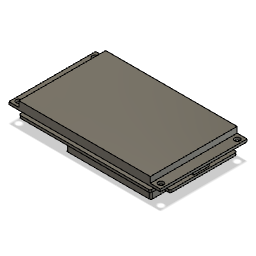
FreeTouchDeck Case V1 (Autodesk Fusion 360 archive; units mm, degrees)
design "ILI9488 TFT"
Autodesk Fusion 360 part; units mm, degrees
sketch "TFT_PCB" plane through (0, 0, 0) normal (0, 1, 0) x (1, 0, 0)
  line L0 (49.15, -28.17) -> (-49.15, -28.17)
  line L1 (-49.15, -28.17) -> (-49.15, 28.17)
  line L2 (-49.15, 28.17) -> (49.15, 28.17)
  line L3 (49.15, 28.17) -> (49.15, -28.17)
  line L4 (49.15, -28.17) -> (-49.15, 28.17) construction
  line L5 (-49.15, -28.17) -> (49.15, 28.17) construction
  line L6 (-42.65, 28.17) -> (-42.65, -28.17)
  line L7 (42.65, 28.17) -> (42.65, -28.17)
  circle A0 centre (-46.15, 24.75) radius 1.75
  line L8 (0, 28.17) -> (0, -28.17) construction
  line L9 (-49.15, 0) -> (49.15, 0) construction
  circle A1 centre (46.15, 24.75) radius 1.75
  circle A2 centre (-46.15, -24.75) radius 1.75
  circle A3 centre (46.15, -24.75) radius 1.75
  dimension "d4" = 98.3
  dimension "d5" = 56.34
  dimension "d6" = 6.5
  dimension "d7" = 6.5
  dimension "d8" = 3.5
  dimension "d9" = 3.42
  dimension "d10" = 3
  constraint horizontal L0
  constraint perpendicular L0 L1
  constraint parallel L0 L2
  constraint parallel L1 L3
  constraint coincident L4 origin
  constraint coincident L5 origin
  constraint coincident L2 L6.start
  constraint coincident L0 L6.end
  constraint perpendicular L0 L6
  constraint coincident L2 L7.start
  constraint coincident L0 L7.end
  constraint perpendicular L0 L7
  constraint midpoint L2 L8.start
  constraint midpoint L0 L8.end
  constraint midpoint L1 L9.start
  constraint midpoint L3 L9.end
  constraint symmetric A0 L8 A1
  constraint symmetric A0 L9 A2
  constraint symmetric L9 A1 A3
  measures "d4" distance of L1.end L2.end
  measures "d5" distance of L0.end L1.end
  measures "d6" distance of L1 L6
  measures "d7" distance of L3 L7
  measures "d8" diameter of A0
  measures "d9" distance of L2 A0.centre
  measures "d10" distance of L1 A0.centre
extrude "Extrude1" add sketch "TFT_PCB" against normal blind 1.6 makes body 1
extrude "Extrude2" add sketch "TFT_PCB" along normal blind 3.79 contours L0 L2 L6 L7 bodies 1
sketch "Sketch2" plane through (0, -1.6, 0) normal (0, -1, 0) x (1, 0, 0)
  circle A0 centre (-46.15, 24.75) radius 1.75
  circle A1 centre (46.15, -24.75) radius 1.75
  circle A2 centre (46.15, 24.75) radius 1.75
  circle A3 centre (-46.15, -24.75) radius 1.75
  line L0 (-49.15, -28.17) -> (49.15, -28.17)
  line L1 (49.15, -28.17) -> (49.15, 28.17)
  line L2 (49.15, 28.17) -> (-49.15, 28.17)
  line L3 (-49.15, 28.17) -> (-49.15, -28.17)
  line L4 (-48.13, 17.69) -> (-45.98, 17.69)
  line L5 (-45.98, 17.69) -> (-45.98, -17.97)
  line L6 (-45.98, -17.97) -> (-48.13, -17.97)
  line L7 (-48.13, -17.97) -> (-48.13, 17.69)
  line L8 (45.98, 5.73) -> (48.13, 5.73)
  line L9 (48.13, 5.73) -> (48.13, -4.67)
  line L10 (48.13, -4.67) -> (45.98, -4.67)
  line L11 (45.98, -4.67) -> (45.98, 5.73)
  dimension "d15" = 2.15
  dimension "d16" = 35.66
  dimension "d17" = 10.2
  dimension "d18" = 1.02
  dimension "d19" = 2.15
  dimension "d20" = 10.4
  dimension "d21" = 1.02
  dimension "d22" = 23.5
  constraint horizontal L4
  constraint vertical L5
  constraint horizontal L6
  constraint vertical L7
  constraint horizontal L8
  constraint vertical L9
  constraint horizontal L10
  constraint vertical L11
  measures "d15" distance of L4.start L4.end
  measures "d16" distance of L4.start L6.end
  measures "d17" distance of L0 L6
  measures "d18" distance of L3 L7
  measures "d19" distance of L8.start L8.end
  measures "d20" distance of L8.start L10.end
  measures "d21" distance of L1 L9
  measures "d22" distance of L0 L10
extrude "Extrude3" add sketch "Sketch2" along normal blind 2.4 contours L4 L5 L6 L7 | L8 L9 L10 L11 bodies 1
sketch "Sketch3" plane through (0, -4, 0) normal (0, -1, 0) x (1, 0, 0)
  line L0 (-48.13, -17.97) -> (-45.98, -17.97)
  line L1 (-45.98, -17.97) -> (-45.98, 17.69)
  line L2 (-45.98, 17.69) -> (-48.13, 17.69)
  line L3 (-48.13, 17.69) -> (-48.13, -17.97)
  line L4 (45.98, -4.67) -> (45.98, 5.73)
  line L5 (45.98, 5.73) -> (48.13, 5.73)
  line L6 (48.13, 5.73) -> (48.13, -4.67)
  line L7 (48.13, -4.67) -> (45.98, -4.67)
  line L8 (-48.13, -17.97) -> (-48.13, 17.69)
  line L9 (-48.13, 17.69) -> (-45.98, 17.69)
  line L10 (-45.98, 17.69) -> (-45.98, -17.97)
  line L11 (-45.98, -17.97) -> (-48.13, -17.97)
  circle A0 centre (-46.15, 24.75) radius 1.75
  circle A1 centre (46.15, -24.75) radius 1.75
  circle A2 centre (46.15, 24.75) radius 1.75
  circle A3 centre (-46.15, -24.75) radius 1.75
  line L12 (-49.15, -28.17) -> (49.15, -28.17)
  line L13 (49.15, -28.17) -> (49.15, 28.17)
  line L14 (49.15, 28.17) -> (-49.15, 28.17)
  line L15 (-49.15, 28.17) -> (-49.15, -28.17)
  line L16 (-49.15, 28.17) -> (-42.65, 28.17)
  line L17 (-42.65, 28.17) -> (-42.65, 21.67)
  line L18 (-42.65, 21.67) -> (-49.15, 21.67)
  line L19 (-49.15, 21.67) -> (-49.15, 28.17)
  line L20 (0, 28.17) -> (0, -28.17) construction
  line L21 (-49.15, 0) -> (49.15, 0) construction
  line L22 (42.65, 28.17) -> (42.65, 21.67)
  line L23 (42.65, 21.67) -> (49.15, 21.67)
  line L24 (42.65, -21.67) -> (49.15, -21.67)
  line L25 (42.65, -28.17) -> (42.65, -21.67)
  line L26 (-42.65, -21.67) -> (-49.15, -21.67)
  line L27 (-42.65, -28.17) -> (-42.65, -21.67)
  line L28 (-15.2668, 24.9101) -> (39.7332, 24.9101)
  line L29 (39.7332, 24.9101) -> (39.7332, -7.0899)
  line L30 (39.7332, -7.0899) -> (-15.2668, -7.0899)
  line L31 (-15.2668, -7.0899) -> (-15.2668, 24.9101)
  dimension "d25" = 6.5
  dimension "d26" = 6.5
  dimension "d27" = 55
  dimension "d28" = 32
  constraint horizontal L16
  constraint vertical L17
  constraint horizontal L18
  constraint vertical L19
  constraint coincident L14.end L15.start
  constraint midpoint L14 L20.start
  constraint midpoint L12 L20.end
  constraint midpoint L15 L21.start
  constraint midpoint L13 L21.end
  constraint symmetric L16.end L20 L22.start
  constraint symmetric L17.end L20 L22.end
  constraint symmetric L18.end L20 L23.end
  constraint symmetric L16.end L21 L27.start
  constraint symmetric L17.end L21 L26.start
  constraint symmetric L18.end L21 L26.end
  constraint symmetric L21 L22.start L25.start
  constraint symmetric L21 L22.end L24.start
  constraint symmetric L21 L23.end L24.end
  constraint horizontal L28
  constraint vertical L29
  constraint horizontal L30
  constraint vertical L31
  measures "d25" distance of L14.end L16.end
  measures "d26" distance of L14.end L18.end
  measures "d27" distance of L28.start L28.end
  measures "d28" distance of L28.start L30.end
extrude "Extrude4" add sketch "Sketch3" along normal blind 1.6 separate body contours L0 L1 L2 L3 L8 L9 L10 L11 | L4 L5 L6 L7 | L12 L13 L14 L15 L17 L18 L22 L23 L24 L25 L26 L27 | L28 L29 L30 L31 makes body 2
extrude "Extrude5" add sketch "Sketch3" along normal blind 8.45 contours L28 L29 L30 L31 bodies 2
fillet "Fillet1" radius 2.5 4 edges at (-42.65, -4.8, 21.67) (-42.65, -4.8, -21.67) (42.65, -4.8, -21.67) (42.65, -4.8, 21.67) on bodies 2
fillet "Fillet2" radius 1 8 edges at (42.65, -4.8, -28.17) (49.15, -4.8, -21.67) (49.15, -4.8, 21.67) (42.65, -4.8, 28.17) (-42.65, -4.8, 28.17) (-49.15, -4.8, 21.67) (-49.15, -4.8, -21.67) (-42.65, -4.8, -28.17) on bodies 2
fillet "Fillet3" radius 1 4 edges at (39.7332, -9.025, 24.9101) (39.7332, -9.025, -7.0899) (-15.2668, -9.025, 24.9101) (-15.2668, -9.025, -7.0899) on bodies 2
equation "pcb_height = 56.34 mm"
equation "pcb_width = 98.3 mm"
equation "d4 = pcb_width"
equation "d5 = pcb_height"
equation "d31 = 1.6 mm + 6.85 mm"
